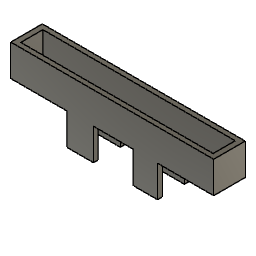
connectorrgb v2 (Autodesk Fusion 360 design; units mm, degrees)
Autodesk Fusion 360 part; units mm, degrees
sketch "Sketch1" plane through (0, 0, 0) normal (0, 0, 1) x (1, 0, 0)
  line L0 (-18.2, 3) -> (78.32, 3)
  line L1 (78.32, 3) -> (78.32, -12)
  line L2 (78.32, -12) -> (-18.2, -12)
  line L3 (-18.2, -12) -> (-18.2, 3)
  line L4 (-18.2, 3) -> (8.47, 3)
  line L5 (8.47, 3) -> (8.47, 0.5)
  line L6 (8.47, 0.5) -> (21.12, 0.5)
  line L7 (21.12, 0.5) -> (21.12, 3)
  line L8 (78.32, 3) -> (51.65, 3)
  line L9 (51.65, 3) -> (39, 3)
  line L10 (39, 3) -> (39, 0.5)
  line L11 (39, 0.5) -> (51.65, 0.5)
  line L12 (51.65, 0.5) -> (51.65, 3)
  line L13 (8.47, -12) -> (21.12, -12)
  line L14 (8.47, -12) -> (8.47, -9.5)
  line L15 (8.47, -9.5) -> (21.12, -9.5)
  line L16 (21.12, -9.5) -> (21.12, -12)
  line L17 (51.65, -12) -> (39, -12)
  line L18 (40, -12) -> (40, -9.5)
  line L19 (51.65, -12) -> (51.65, -9.5)
  line L20 (40, -9.5) -> (51.65, -9.5)
  dimension "d1" = 96.52
  dimension "d2" = 15
  dimension "d3" = 26.67
  dimension "d4" = 2.5
  dimension "d5" = 12.65
  dimension "d6" = 26.67
  dimension "d7" = 12.65
  dimension "d8" = 12.65
  dimension "d9" = 2.5
  dimension "d10" = 12.65
  dimension "d11" = 2.5
  dimension "d12" = 2.5
  constraint horizontal L0
  constraint vertical L1
  constraint horizontal L2
  constraint vertical L3
  constraint coincident L0 L4.end
  constraint perpendicular L0 L5
  constraint perpendicular L5 L6
  constraint coincident L0 L7.end
  constraint perpendicular L0 L7
  constraint perpendicular L1 L8
  constraint horizontal L9
  constraint vertical L10
  constraint horizontal L11
  constraint vertical L12
  constraint coincident L2 L13.start
  constraint coincident L2 L13.end
  constraint perpendicular L13 L14
  constraint perpendicular L14 L15
  constraint coincident L2 L17.start
  constraint coincident L2 L17.end
  constraint perpendicular L12 L17
  constraint coincident L2 L18.start
  constraint perpendicular L2 L18
  constraint perpendicular L17 L19
  measures "d1" distance of L0.start L0.end
  measures "d2" distance of L0.start L2.end
  measures "d3" distance of L0.start L4.end
  measures "d4" distance of L4.end L5.end
  measures "d5" distance of L5.end L6.end
  measures "d6" distance of L0.end L8.end
  measures "d7" distance of L8.end L9.end
  measures "d8" distance of L13.start L13.end
  measures "d9" distance of L13.start L14.end
  measures "d10" distance of L14.end L15.end
  measures "d11" distance of L18.start L18.end
  measures "d12" distance of L17.start L19.end
extrude "Extrude1" add sketch "Sketch1" along normal blind 15 contours L0 L1 L2 L3 L4 L5 L6 L7 L8 L10 L11 L12 L14 L15 L16 L17 L18 L19 L20 makes body 1
sketch "Sketch2" plane through (0, 0, 0) normal (0, 0, -1) x (1, 0, 0)
  line L0 (40, 9.5) -> (40, 12)
  line L1 (40, 12) -> (21.12, 12)
  line L2 (21.12, 12) -> (21.12, 9.5)
  line L3 (21.12, 9.5) -> (8.47, 9.5)
  line L4 (8.47, 9.5) -> (8.47, 12)
  line L5 (8.47, 12) -> (-18.2, 12)
  line L6 (-18.2, 12) -> (-18.2, -3)
  line L7 (-18.2, -3) -> (8.47, -3)
  line L8 (8.47, -3) -> (8.47, -0.5)
  line L9 (8.47, -0.5) -> (21.12, -0.5)
  line L10 (21.12, -0.5) -> (21.12, -3)
  line L11 (21.12, -3) -> (39, -3)
  line L12 (39, -3) -> (39, -0.5)
  line L13 (39, -0.5) -> (51.65, -0.5)
  line L14 (51.65, -0.5) -> (51.65, -3)
  line L15 (51.65, -3) -> (78.32, -3)
  line L16 (78.32, -3) -> (78.32, 12)
  line L17 (78.32, 12) -> (51.65, 12)
  line L18 (51.65, 12) -> (51.65, 9.5)
  line L19 (51.65, 9.5) -> (40, 9.5)
  line L20 (8.47, 12) -> (21.12, 12)
  line L21 (21.12, 12) -> (21.12, 9.5)
  line L22 (21.12, 9.5) -> (8.47, 9.5)
  line L23 (8.47, 9.5) -> (8.47, 12)
  line L24 (8.47, -0.5) -> (21.12, -0.5)
  line L25 (21.12, -0.5) -> (21.12, -3)
  line L26 (21.12, -3) -> (8.47, -3)
  line L27 (8.47, -3) -> (8.47, -0.5)
  line L28 (40, 12) -> (51.65, 12)
  line L29 (51.65, 12) -> (51.65, 9.5)
  line L30 (51.65, 9.5) -> (40, 9.5)
  line L31 (40, 9.5) -> (40, 12)
  line L32 (39, -0.5) -> (51.65, -0.5)
  line L33 (51.65, -0.5) -> (51.65, -3)
  line L34 (51.65, -3) -> (39, -3)
  line L35 (39, -3) -> (39, -0.5)
  constraint horizontal L20
  constraint vertical L21
  constraint horizontal L22
  constraint vertical L23
  constraint coincident L2.end L3.start
  constraint coincident L4.end L5.start
  constraint horizontal L24
  constraint vertical L25
  constraint horizontal L26
  constraint vertical L27
  constraint coincident L10.end L11.start
  constraint coincident L8.end L9.start
  constraint horizontal L28
  constraint vertical L29
  constraint horizontal L30
  constraint vertical L31
  constraint coincident L18.end L19.start
  constraint coincident L0.end L1.start
  constraint horizontal L32
  constraint vertical L33
  constraint horizontal L34
  constraint vertical L35
  constraint coincident L14.end L15.start
  constraint coincident L12.end L13.start
extrude "Extrude2" add sketch "Sketch2" along normal blind 15 separate body contours L0 L18 L19 L28 L29 L30 L31 | L2 L3 L4 L20 L21 L22 L23 | L12 L13 L14 L32 L33 L34 L35 | L8 L9 L10 L24 L25 L26 L27 makes body 2 at (47.7667, -9.5, -5) makes body 3 at (47.4333, 3, -5) makes body 4 at (16.9033, -9.5, -5) makes body 5 at (12.6867, 0.5, -5)
extrude "Extrude3" add 4 faces at (43.2167, 1.3333, 0) (12.6867, 1.3333, 0) (16.9033, -11.1667, 0) (47.7667, -10.3333, 0) along direction (0, 0, 1) blind 15 on bodies 2 3 4 5 bodies 1 3 2 4 5
sketch "Sketch3" plane through (0, 0, 15) normal (0, 0, 1) x (-1, 0, 0)
  line L0 (18.2, 12) -> (-78.32, 12)
  line L1 (-78.32, 12) -> (-78.32, -3)
  line L2 (-78.32, -3) -> (18.2, -3)
  line L3 (18.2, -3) -> (18.2, 12)
  line L4 (-75.82, 9.75) -> (15.7, 9.75)
  line L5 (15.7, 9.75) -> (15.7, -0.75)
  line L6 (15.7, -0.75) -> (-75.82, -0.75)
  line L7 (-75.82, -0.75) -> (-75.82, 9.75)
  line L8 (-78.32, 12) -> (-75.82, 12)
  line L9 (-75.82, 12) -> (-75.82, 9.75)
  dimension "d19" = 91.52
  dimension "d20" = 10.5
  dimension "d21" = 2.5
  dimension "d22" = 2.25
  constraint horizontal L4
  constraint vertical L5
  constraint horizontal L6
  constraint vertical L7
  constraint coincident L0.end L1.start
  constraint perpendicular L1 L8
  constraint perpendicular L8 L9
  measures "d19" distance of L4.end L4.start
  measures "d20" distance of L6.end L4.start
  measures "d21" distance of L0.end L8.end
  measures "d22" distance of L8.end L4.start
extrude "Extrude4" cut sketch "Sketch3" against normal blind 12.5 contours L4 L5 L6 L7 bodies 1
sketch "Sketch4" plane through (0, 0, 2.5) normal (0, 0, 1) x (-1, 0, 0)
  line L0 (-75.82, -0.75) -> (15.7, -0.75)
  line L1 (15.7, -0.75) -> (15.7, 9.75)
  line L2 (15.7, 9.75) -> (-75.82, 9.75)
  line L3 (-75.82, 9.75) -> (-75.82, -0.75)
  line L4 (-75.82, 4.5) -> (-70.7, 4.5)
  circle A0 centre (-70.7, 4.5) radius 1.6
  line L5 (15.7, 4.5) -> (10.58, 4.5)
  circle A1 centre (10.58, 4.5) radius 1.6
  dimension "d25" = 5.12
  dimension "d26" = 3.2
  dimension "d27" = 5.12
  dimension "d28" = 3.2
  constraint midpoint L3 L4.start
  constraint perpendicular L3 L4
  constraint coincident L4.end A0.centre
  constraint midpoint L1 L5.start
  constraint perpendicular L1 L5
  constraint coincident L5.end A1.centre
  measures "d25" distance of L4.start L4.end
  measures "d26" diameter of A0
  measures "d27" distance of L5.start L5.end
  measures "d28" diameter of A1
extrude "Extrude5" cut sketch "Sketch4" against normal blind 100 contours A0 | A1 bodies 1
sketch "Sketch5" plane through (0, 0, 2.5) normal (0, 0, 1) x (-1, 0, 0)
  circle A0 centre (10.58, 4.5) radius 1.6
  circle A1 centre (-70.7, 4.5) radius 1.6
  line L0 (-75.82, -0.75) -> (15.7, -0.75)
  line L1 (15.7, -0.75) -> (15.7, 9.75)
  line L2 (15.7, 9.75) -> (-75.82, 9.75)
  line L3 (-75.82, 9.75) -> (-75.82, -0.75)
  circle A2 centre (10.58, 4.5) radius 3.5
  circle A3 centre (-70.7, 4.5) radius 3.5
  dimension "d31" = 7
  dimension "d32" = 7
  constraint concentric A0 A2
  constraint concentric A1 A3
  measures "d31" diameter of A2
  measures "d32" diameter of A3
extrude "Extrude6" cut sketch "Sketch5" against normal blind 1 contours A2 | A3 bodies 1
sketch "Sketch6" plane through (0, 0, 2.5) normal (0, 0, 1) x (-1, 0, 0)
  circle A0 centre (-70.7, 4.5) radius 3.5
  circle A1 centre (10.58, 4.5) radius 3.5
  line L0 (-75.82, -0.75) -> (15.7, -0.75)
  line L1 (15.7, -0.75) -> (15.7, 9.75)
  line L2 (15.7, 9.75) -> (-75.82, 9.75)
  line L3 (-75.82, 9.75) -> (-75.82, -0.75)
  line L4 (-75.82, 4.5) -> (-78.3, 4.5)
  line L5 (-75.82, 4.5) -> (-51.65, 4.5)
  line L6 (-51.65, 4.5) -> (-38.95, 4.5)
  line L7 (15.7, 4.5) -> (-8.47, 4.5)
  line L8 (-8.47, 4.5) -> (-21.17, 4.5)
  line L9 (-38.95, 9.75) -> (-51.65, 9.75)
  line L10 (-51.65, 9.75) -> (-51.65, -0.75)
  line L11 (-51.65, -0.75) -> (-38.95, -0.75)
  line L12 (-38.95, -0.75) -> (-38.95, 9.75)
  line L13 (-8.47, -0.75) -> (-21.17, -0.75)
  line L14 (-21.17, -0.75) -> (-21.17, 9.75)
  line L15 (-21.17, 9.75) -> (-8.47, 9.75)
  line L16 (-8.47, 9.75) -> (-8.47, -0.75)
  dimension "d35" = 24.17
  dimension "d36" = 12.7
  dimension "d37" = 24.17
  dimension "d38" = 12.7
  constraint midpoint L3 L4.start
  constraint perpendicular L3 L4
  constraint perpendicular L3 L5
  constraint parallel L5 L6
  constraint midpoint L1 L7.start
  constraint perpendicular L1 L7
  constraint perpendicular L1 L8
  constraint horizontal L9
  constraint vertical L10
  constraint horizontal L11
  constraint vertical L12
  constraint coincident L0 L10.end
  constraint coincident L2 L9.start
  constraint horizontal L13
  constraint vertical L14
  constraint horizontal L15
  constraint vertical L16
  constraint coincident L2 L14.end
  constraint coincident L0 L13.start
  measures "d35" distance of L4.start L5.end
  measures "d36" distance of L5.end L6.end
  measures "d37" distance of L7.start L7.end
  measures "d38" distance of L7.end L8.end
extrude "Extrude7" cut sketch "Sketch6" against normal blind 100 contours L2 L6 L9 L10 L12 | L0 L6 L10 L11 L12 | L0 L8 L13 L14 L16 | L2 L8 L14 L15 L16 bodies 1
